Autodesk Fusion 360 part; units mm, degrees
note: some values were not read from the file. Set by a fixed rule: which sketch regions a step uses.
(part 2 of 3)
  arc A385 (-20.318, -125.058) -> (-9.818, -135.558) centre (-9.818, -125.058) ccw
  line L386 (-9.818, -135.558) -> (410.182, -135.558)
  arc A386 (410.182, -135.558) -> (420.682, -125.058) centre (410.182, -125.058) ccw
  line L387 (420.682, -125.058) -> (420.682, 4.942)
  arc A387 (420.682, 4.942) -> (410.182, 15.442) centre (410.182, 4.942) ccw
  line L388 (-20.318, 4.692) -> (-22.818, 4.692)
  line L389 (-23.818, 3.692) -> (-23.818, -4.308)
  line L390 (-22.818, -5.308) -> (-20.318, -5.308)
  line L391 (-20.318, -5.308) -> (-20.318, 4.692)
  arc A388 (-22.818, 4.692) -> (-23.818, 3.692) centre (-22.818, 3.692) ccw
  arc A389 (-23.818, -4.308) -> (-22.818, -5.308) centre (-22.818, -4.308) ccw
  line L392 (-23.818, -26.183) -> (-23.818, -34.183)
  line L393 (-20.318, -25.183) -> (-22.818, -25.183)
  line L394 (-22.818, -35.183) -> (-20.318, -35.183)
  arc A390 (-23.818, -34.183) -> (-22.818, -35.183) centre (-22.818, -34.183) ccw
  arc A391 (-22.818, -25.183) -> (-23.818, -26.183) centre (-22.818, -26.183) ccw
  line L395 (-23.818, -56.058) -> (-23.818, -64.058)
  line L396 (-20.318, -55.058) -> (-22.818, -55.058)
  line L397 (-22.818, -65.058) -> (-20.318, -65.058)
  arc A392 (-23.818, -64.058) -> (-22.818, -65.058) centre (-22.818, -64.058) ccw
  arc A393 (-22.818, -55.058) -> (-23.818, -56.058) centre (-22.818, -56.058) ccw
  line L398 (-23.818, -85.933) -> (-23.818, -93.933)
  line L399 (-20.318, -84.933) -> (-22.818, -84.933)
  line L400 (-22.818, -94.933) -> (-20.318, -94.933)
  arc A394 (-23.818, -93.933) -> (-22.818, -94.933) centre (-22.818, -93.933) ccw
  arc A395 (-22.818, -84.933) -> (-23.818, -85.933) centre (-22.818, -85.933) ccw
  line L401 (-23.818, -115.808) -> (-23.818, -123.808)
  line L402 (-20.318, -114.808) -> (-22.818, -114.808)
  line L403 (-22.818, -124.808) -> (-20.318, -124.808)
  arc A396 (-23.818, -123.808) -> (-22.818, -124.808) centre (-22.818, -123.808) ccw
  arc A397 (-22.818, -114.808) -> (-23.818, -115.808) centre (-22.818, -115.808) ccw
  line L404 (420.682, 4.692) -> (423.182, 4.692)
  line L405 (424.182, 3.692) -> (424.182, -4.308)
  line L406 (423.182, -5.308) -> (420.682, -5.308)
  line L407 (420.682, -5.308) -> (420.682, 4.692)
  arc A398 (424.182, 3.692) -> (423.182, 4.692) centre (423.182, 3.692) ccw
  arc A399 (423.182, -5.308) -> (424.182, -4.308) centre (423.182, -4.308) ccw
  arc A400 (423.182, -65.058) -> (424.182, -64.058) centre (423.182, -64.058) ccw
  line L408 (423.182, -65.058) -> (420.682, -65.058)
  line L409 (424.182, -56.058) -> (424.182, -64.058)
  line L410 (420.682, -55.058) -> (423.182, -55.058)
  arc A401 (424.182, -56.058) -> (423.182, -55.058) centre (423.182, -56.058) ccw
  arc A402 (423.182, -94.933) -> (424.182, -93.933) centre (423.182, -93.933) ccw
  line L411 (423.182, -94.933) -> (420.682, -94.933)
  line L412 (424.182, -85.933) -> (424.182, -93.933)
  line L413 (420.682, -84.933) -> (423.182, -84.933)
  arc A403 (424.182, -85.933) -> (423.182, -84.933) centre (423.182, -85.933) ccw
  line L414 (-9.568, 15.442) -> (0.432, 15.442)
  line L415 (0.432, 15.442) -> (0.432, 17.942)
  line L416 (-0.568, 18.942) -> (-8.568, 18.942)
  line L417 (-9.568, 17.942) -> (-9.568, 15.442)
  arc A404 (-8.568, 18.942) -> (-9.568, 17.942) centre (-8.568, 17.942) ccw
  arc A405 (0.432, 17.942) -> (-0.568, 18.942) centre (-0.568, 17.942) ccw
  line L418 (41.6195, 17.942) -> (41.6195, 15.442)
  arc A406 (42.6195, 18.942) -> (41.6195, 17.942) centre (42.6195, 17.942) ccw
  line L419 (50.6195, 18.942) -> (42.6195, 18.942)
  line L420 (51.6195, 15.442) -> (51.6195, 17.942)
  arc A407 (51.6195, 17.942) -> (50.6195, 18.942) centre (50.6195, 17.942) ccw
  line L421 (92.807, 17.942) -> (92.807, 15.442)
  arc A408 (93.807, 18.942) -> (92.807, 17.942) centre (93.807, 17.942) ccw
  line L422 (101.807, 18.942) -> (93.807, 18.942)
  line L423 (102.807, 15.442) -> (102.807, 17.942)
  arc A409 (102.807, 17.942) -> (101.807, 18.942) centre (101.807, 17.942) ccw
  line L424 (143.9945, 17.942) -> (143.9945, 15.442)
  arc A410 (144.9945, 18.942) -> (143.9945, 17.942) centre (144.9945, 17.942) ccw
  line L425 (152.9945, 18.942) -> (144.9945, 18.942)
  line L426 (153.9945, 15.442) -> (153.9945, 17.942)
  arc A411 (153.9945, 17.942) -> (152.9945, 18.942) centre (152.9945, 17.942) ccw
  line L427 (195.182, 17.942) -> (195.182, 15.442)
  arc A412 (196.182, 18.942) -> (195.182, 17.942) centre (196.182, 17.942) ccw
  line L428 (204.182, 18.942) -> (196.182, 18.942)
  line L429 (205.182, 15.442) -> (205.182, 17.942)
  arc A413 (205.182, 17.942) -> (204.182, 18.942) centre (204.182, 17.942) ccw
  line L430 (246.3695, 17.942) -> (246.3695, 15.442)
  arc A414 (247.3695, 18.942) -> (246.3695, 17.942) centre (247.3695, 17.942) ccw
  line L431 (255.3695, 18.942) -> (247.3695, 18.942)
  line L432 (256.3695, 15.442) -> (256.3695, 17.942)
  arc A415 (256.3695, 17.942) -> (255.3695, 18.942) centre (255.3695, 17.942) ccw
  line L433 (297.557, 17.942) -> (297.557, 15.442)
  arc A416 (298.557, 18.942) -> (297.557, 17.942) centre (298.557, 17.942) ccw
  line L434 (306.557, 18.942) -> (298.557, 18.942)
  line L435 (307.557, 15.442) -> (307.557, 17.942)
  arc A417 (307.557, 17.942) -> (306.557, 18.942) centre (306.557, 17.942) ccw
  line L436 (348.7445, 17.942) -> (348.7445, 15.442)
  arc A418 (349.7445, 18.942) -> (348.7445, 17.942) centre (349.7445, 17.942) ccw
  line L437 (357.7445, 18.942) -> (349.7445, 18.942)
  line L438 (358.7445, 15.442) -> (358.7445, 17.942)
  arc A419 (358.7445, 17.942) -> (357.7445, 18.942) centre (357.7445, 17.942) ccw
  line L439 (399.932, 17.942) -> (399.932, 15.442)
  arc A420 (400.932, 18.942) -> (399.932, 17.942) centre (400.932, 17.942) ccw
  line L440 (408.932, 18.942) -> (400.932, 18.942)
  line L441 (409.932, 15.442) -> (409.932, 17.942)
  arc A421 (409.932, 17.942) -> (408.932, 18.942) centre (408.932, 17.942) ccw
  line L442 (-9.568, -139.4053) -> (-9.818, -139.4053)
  line L443 (-9.568, -135.558) -> (0.432, -135.558)
  line L444 (0.432, -135.558) -> (0.432, -138.058)
  line L445 (-0.568, -139.058) -> (-8.568, -139.058)
  line L446 (-9.568, -138.058) -> (-9.568, -135.558)
  arc A422 (-9.568, -138.058) -> (-8.568, -139.058) centre (-8.568, -138.058) ccw
  arc A423 (-0.568, -139.058) -> (0.432, -138.058) centre (-0.568, -138.058) ccw
  line L447 (41.6195, -138.058) -> (41.6195, -135.558)
  arc A424 (41.6195, -138.058) -> (42.6195, -139.058) centre (42.6195, -138.058) ccw
  line L448 (50.6195, -139.058) -> (42.6195, -139.058)
  arc A425 (50.6195, -139.058) -> (51.6195, -138.058) centre (50.6195, -138.058) ccw
  line L449 (51.6195, -135.558) -> (51.6195, -138.058)
  line L450 (92.807, -138.058) -> (92.807, -135.558)
  arc A426 (92.807, -138.058) -> (93.807, -139.058) centre (93.807, -138.058) ccw
  line L451 (101.807, -139.058) -> (93.807, -139.058)
  arc A427 (101.807, -139.058) -> (102.807, -138.058) centre (101.807, -138.058) ccw
  line L452 (102.807, -135.558) -> (102.807, -138.058)
  line L453 (143.9945, -138.058) -> (143.9945, -135.558)
  arc A428 (143.9945, -138.058) -> (144.9945, -139.058) centre (144.9945, -138.058) ccw
  line L454 (152.9945, -139.058) -> (144.9945, -139.058)
  arc A429 (152.9945, -139.058) -> (153.9945, -138.058) centre (152.9945, -138.058) ccw
  line L455 (153.9945, -135.558) -> (153.9945, -138.058)
  line L456 (195.182, -138.058) -> (195.182, -135.558)
  arc A430 (195.182, -138.058) -> (196.182, -139.058) centre (196.182, -138.058) ccw
  line L457 (204.182, -139.058) -> (196.182, -139.058)
  arc A431 (204.182, -139.058) -> (205.182, -138.058) centre (204.182, -138.058) ccw
  line L458 (205.182, -135.558) -> (205.182, -138.058)
  line L459 (246.3695, -138.058) -> (246.3695, -135.558)
  arc A432 (246.3695, -138.058) -> (247.3695, -139.058) centre (247.3695, -138.058) ccw
  line L460 (255.3695, -139.058) -> (247.3695, -139.058)
  arc A433 (255.3695, -139.058) -> (256.3695, -138.058) centre (255.3695, -138.058) ccw
  line L461 (256.3695, -135.558) -> (256.3695, -138.058)
  line L462 (297.557, -138.058) -> (297.557, -135.558)
  arc A434 (297.557, -138.058) -> (298.557, -139.058) centre (298.557, -138.058) ccw
  line L463 (306.557, -139.058) -> (298.557, -139.058)
  arc A435 (306.557, -139.058) -> (307.557, -138.058) centre (306.557, -138.058) ccw
  line L464 (307.557, -135.558) -> (307.557, -138.058)
  line L465 (348.7445, -138.058) -> (348.7445, -135.558)
  arc A436 (348.7445, -138.058) -> (349.7445, -139.058) centre (349.7445, -138.058) ccw
  line L466 (357.7445, -139.058) -> (349.7445, -139.058)
  arc A437 (357.7445, -139.058) -> (358.7445, -138.058) centre (357.7445, -138.058) ccw
  line L467 (358.7445, -135.558) -> (358.7445, -138.058)
  line L468 (399.932, -138.058) -> (399.932, -135.558)
  arc A438 (399.932, -138.058) -> (400.932, -139.058) centre (400.932, -138.058) ccw
  line L469 (408.932, -139.058) -> (400.932, -139.058)
  arc A439 (408.932, -139.058) -> (409.932, -138.058) centre (408.932, -138.058) ccw
  line L470 (409.932, -135.558) -> (409.932, -138.058)
  arc A440 (373.352, -130.228) -> (376.152, -127.428) centre (373.352, -127.428) ccw
  line L471 (376.152, -125.488) -> (376.152, -127.428)
  arc A441 (376.152, -125.488) -> (373.352, -122.688) centre (373.352, -125.488) ccw
  line L472 (348.552, -122.688) -> (373.352, -122.688)
  arc A442 (348.552, -122.688) -> (345.752, -125.488) centre (348.552, -125.488) ccw
  line L473 (345.752, -127.428) -> (345.752, -125.488)
  arc A443 (345.752, -127.428) -> (348.552, -130.228) centre (348.552, -127.428) ccw
  line L474 (373.352, -130.228) -> (348.552, -130.228)
  arc A444 (395.862, -124.298) -> (394.562, -125.598) centre (395.862, -125.598) ccw
  line L475 (394.562, -130.078) -> (394.562, -125.598)
  arc A445 (394.562, -130.078) -> (395.862, -131.378) centre (395.862, -130.078) ccw
  line L476 (397.802, -131.378) -> (395.862, -131.378)
  arc A446 (397.802, -131.378) -> (399.102, -130.078) centre (397.802, -130.078) ccw
  line L477 (399.102, -125.598) -> (399.102, -130.078)
  arc A447 (399.102, -125.598) -> (397.802, -124.298) centre (397.802, -125.598) ccw
  line L478 (395.862, -124.298) -> (397.802, -124.298)
  arc A448 (383.062, -9.148) -> (381.762, -7.848) centre (381.762, -9.148) ccw
  line L479 (367.122, -7.848) -> (381.762, -7.848)
  arc A449 (367.122, -7.848) -> (365.822, -9.148) centre (367.122, -9.148) ccw
  line L480 (365.822, -13.628) -> (365.822, -9.148)
  arc A450 (365.822, -13.628) -> (367.122, -14.928) centre (367.122, -13.628) ccw
  line L481 (381.762, -14.928) -> (367.122, -14.928)
  arc A451 (381.762, -14.928) -> (383.062, -13.628) centre (381.762, -13.628) ccw
  line L482 (383.062, -9.148) -> (383.062, -13.628)
  line L483 (411.977, -14.103) -> (397.337, -14.103)
  line L484 (396.037, -12.803) -> (396.037, -10.863)
  line L485 (397.337, -9.563) -> (411.977, -9.563)
  arc A452 (396.037, -12.803) -> (397.337, -14.103) centre (397.337, -12.803) ccw
  arc A453 (397.337, -9.563) -> (396.037, -10.863) centre (397.337, -10.863) ccw
  arc A454 (411.977, -14.103) -> (413.277, -12.803) centre (411.977, -12.803) ccw
  line L486 (413.277, -10.863) -> (413.277, -12.803)
  arc A455 (413.277, -10.863) -> (411.977, -9.563) centre (411.977, -10.863) ccw
  arc A456 (412.123, 3.662) -> (410.823, 4.962) centre (410.823, 3.662) ccw
  line L487 (406.143, 4.962) -> (410.823, 4.962)
  arc A457 (406.143, 4.962) -> (404.843, 3.662) centre (406.143, 3.662) ccw
  line L488 (404.843, 1.722) -> (404.843, 3.662)
  arc A458 (404.843, 1.722) -> (406.143, 0.422) centre (406.143, 1.722) ccw
  line L489 (410.823, 0.422) -> (406.143, 0.422)
  arc A459 (410.823, 0.422) -> (412.123, 1.722) centre (410.823, 1.722) ccw
  line L490 (412.123, 3.662) -> (412.123, 1.722)
  point P0 (-23.818, 4.692)
  point P1 (424.182, 4.692)
  point P2 (-9.568, 18.942)
  point P3 (-9.568, -139.058)
  dimension "d12" = 3.5
  dimension "d13" = 10
  dimension "d14" = 1
  dimension "d17" = 0
  dimension "d18" = -119.5
  dimension "d23" = 3.5
  dimension "d24" = 10
  dimension "d25" = 1
  dimension "d28" = 0
  dimension "d29" = -119.5
  dimension "d31" = 10
  dimension "d32" = 3.5
  dimension "d33" = 1
  dimension "d36" = 409.5
  dimension "d37" = 0
  dimension "d39" = 10
  dimension "d40" = 3.5
  dimension "d41" = 1
  dimension "d44" = 409.5
  dimension "d45" = 0
  constraint horizontal L388
  constraint vertical L389
  constraint horizontal L390
  constraint vertical L391
  constraint coincident P0 L388
  constraint coincident P0 L389
  constraint tangent L388 A388
  constraint tangent L389 A388
  constraint tangent L390 A389
  constraint tangent L389 A389
  constraint equal A388 A389
  constraint horizontal L404
  constraint vertical L405
  constraint horizontal L406
  constraint vertical L407
  constraint coincident P1 L404
  constraint coincident P1 L405
  constraint tangent L404 A398
  constraint tangent L405 A398
  constraint tangent L405 A399
  constraint tangent L406 A399
  constraint equal A398 A399
  constraint horizontal L414
  constraint vertical L415
  constraint horizontal L416
  constraint vertical L417
  constraint coincident P2 L417
  constraint coincident P2 L416
  constraint tangent L417 A404
  constraint tangent L416 A404
  constraint tangent L415 A405
  constraint tangent L416 A405
  constraint equal A404 A405
  constraint horizontal L442
  constraint horizontal L443
  constraint vertical L444
  constraint horizontal L445
  constraint vertical L446
  constraint coincident P3 L446
  constraint coincident P3 L445
  constraint tangent L446 A422
  constraint tangent L445 A422
  constraint tangent L445 A423
  constraint tangent L444 A423
  constraint equal A422 A423
  measures "d12" distance of L388.start P0
  measures "d13" distance of L388.start L390.end
  measures "d14" radius of A388
  measures "d23" distance of L404.start P1
  measures "d24" distance of L404.start L406.end
  measures "d25" radius of A398
  measures "d31" distance of L414.start L414.end
  measures "d32" distance of L414.start P2
  measures "d33" radius of A404
  measures "d39" distance of L443.start L443.end
  measures "d40" distance of L443.start P3
  measures "d41" radius of A422
extrude "Extrude1" add sketch "Sketch1" along normal blind 1.5 contours L384 A384 L385 A385 L386 A386 L387 A387 L391 L407 L414 L443 | A440 L471 A441 L472 A442 L473 A443 L474 | A444 L475 A445 L476 A446 L477 A447 L478 | A448 L479 A449 L480 A450 L481 A451 L482 | L483 L484 L485 A452 A453 A454 L486 A455 | A456 L487 A457 L488 A458 L489 A459 L490
extrude "Extrude2" add sketch "Sketch1" along normal blind 1.5 contours L385 L388 L389 L390 L391 A388 A389 | L385 L392 L393 L394 A390 A391 | L385 L395 L396 L397 A392 A393 | L385 L398 L399 L400 A394 A395 | L385 L401 L402 L403 A396 A397
extrude "Extrude3" add sketch "Sketch1" along normal blind 1.5 contours L384 L439 A420 L440 L441 A421 | L387 L404 L405 L406 L407 A398 A399 | L384 L436 A418 L437 L438 A419 | L387 A400 L408 L409 L410 A401 | L384 L433 A416 L434 L435 A417 | L387 A402 L411 L412 L413 A403 | L384 L430 A414 L431 L432 A415 | L384 L427 A412 L428 L429 A413 | L386 L468 A438 L469 A439 L470 | L384 L424 A410 L425 L426 A411 | L386 L465 A436 L466 A437 L467 | L384 L421 A408 L422 L423 A409 | L386 L462 A434 L463 A435 L464 | L384 L418 A406 L419 L420 A407 | L386 L459 A432 L460 A433 L461 | L384 L414 L415 L416 L417 A404 A405 | L386 L456 A430 L457 A431 L458 | L386 L453 A428 L454 A429 L455 | L386 L450 A426 L451 A427 L452 | L386 L447 A424 L448 A425 L449 | L386 L443 L444 L445 L446 A422 A423
extrude "Extrude4" cut sketch "Sketch1" along normal blind 3 contours A440 L471 A441 L472 A442 L473 A443 L474
extrude "Extrude5" cut sketch "Sketch1" along normal blind 2 contours A444 L475 A445 L476 A446 L477 A447 L478
extrude "Extrude6" cut sketch "Sketch1" along normal blind 10 contours A448 L479 A449 L480 A450 L481 A451 L482
extrude "Extrude7" cut sketch "Sketch1" along normal blind 15 contours L483 L484 L485 A452 A453 A454 L486 A455
extrude "Extrude8" cut sketch "Sketch1" along normal blind 5 contours A456 L487 A457 L488 A458 L489 A459 L490
sketch "Sketch3" plane through (0, 0, 1.5) normal (0, 0, 1) x (-1, 0, 0)
  line L0 (-406.143, -4.962) -> (-410.823, -4.962)
  arc A0 (-412.123, -3.662) -> (-410.823, -4.962) centre (-410.823, -3.662) ccw
  line L1 (-412.123, -3.662) -> (-412.123, -1.722)
  arc A1 (-410.823, -0.422) -> (-412.123, -1.722) centre (-410.823, -1.722) ccw
  line L2 (-410.823, -0.422) -> (-406.143, -0.422)
  arc A2 (-404.843, -1.722) -> (-406.143, -0.422) centre (-406.143, -1.722) ccw
  line L3 (-404.843, -1.722) -> (-404.843, -3.662)
  arc A3 (-406.143, -4.962) -> (-404.843, -3.662) centre (-406.143, -3.662) ccw
  line L4 (-411.977, 14.103) -> (-397.337, 14.103)
  arc A4 (-396.037, 12.803) -> (-397.337, 14.103) centre (-397.337, 12.803) ccw
  line L5 (-396.037, 12.803) -> (-396.037, 10.863)
  arc A5 (-397.337, 9.563) -> (-396.037, 10.863) centre (-397.337, 10.863) ccw
  line L6 (-397.337, 9.563) -> (-411.977, 9.563)
  arc A6 (-413.277, 10.863) -> (-411.977, 9.563) centre (-411.977, 10.863) ccw
  line L7 (-413.277, 10.863) -> (-413.277, 12.803)
  arc A7 (-411.977, 14.103) -> (-413.277, 12.803) centre (-411.977, 12.803) ccw
  line L8 (-367.122, 7.848) -> (-381.762, 7.848)
  arc A8 (-383.062, 9.148) -> (-381.762, 7.848) centre (-381.762, 9.148) ccw
  line L9 (-383.062, 9.148) -> (-383.062, 13.628)
  arc A9 (-381.762, 14.928) -> (-383.062, 13.628) centre (-381.762, 13.628) ccw
  line L10 (-381.762, 14.928) -> (-367.122, 14.928)
  arc A10 (-365.822, 13.628) -> (-367.122, 14.928) centre (-367.122, 13.628) ccw
  line L11 (-365.822, 13.628) -> (-365.822, 9.148)
  arc A11 (-367.122, 7.848) -> (-365.822, 9.148) centre (-367.122, 9.148) ccw
  line L12 (-394.562, 130.078) -> (-394.562, 125.598)
  arc A12 (-395.862, 124.298) -> (-394.562, 125.598) centre (-395.862, 125.598) ccw
  line L13 (-395.862, 124.298) -> (-397.802, 124.298)
  arc A13 (-399.102, 125.598) -> (-397.802, 124.298) centre (-397.802, 125.598) ccw
  line L14 (-399.102, 125.598) -> (-399.102, 130.078)
  arc A14 (-397.802, 131.378) -> (-399.102, 130.078) centre (-397.802, 130.078) ccw
  line L15 (-397.802, 131.378) -> (-395.862, 131.378)
  arc A15 (-394.562, 130.078) -> (-395.862, 131.378) centre (-395.862, 130.078) ccw
  line L16 (-376.152, 125.488) -> (-376.152, 127.428)
  arc A16 (-373.352, 130.228) -> (-376.152, 127.428) centre (-373.352, 127.428) ccw
  line L17 (-373.352, 130.228) -> (-348.552, 130.228)
  arc A17 (-345.752, 127.428) -> (-348.552, 130.228) centre (-348.552, 127.428) ccw
  line L18 (-345.752, 127.428) -> (-345.752, 125.488)
  arc A18 (-348.552, 122.688) -> (-345.752, 125.488) centre (-348.552, 125.488) ccw
  line L19 (-348.552, 122.688) -> (-373.352, 122.688)
  arc A19 (-376.152, 125.488) -> (-373.352, 122.688) centre (-373.352, 125.488) ccw
  arc A20 (-50.65, 50.15) -> (-50.15, 50.65) centre (-50.65, 50.65) ccw
  line L20 (-50.65, 50.15) -> (-63.65, 50.15)
  arc A21 (-64.15, 50.65) -> (-63.65, 50.15) centre (-63.65, 50.65) ccw
  line L21 (-64.15, 50.65) -> (-64.15, 63.65)
  arc A22 (-63.65, 64.15) -> (-64.15, 63.65) centre (-63.65, 63.65) ccw
  line L22 (-63.65, 64.15) -> (-50.65, 64.15)
  arc A23 (-50.15, 63.65) -> (-50.65, 64.15) centre (-50.65, 63.65) ccw
  line L23 (-50.15, 63.65) -> (-50.15, 50.65)
  arc A24 (-203.05, 50.15) -> (-202.55, 50.65) centre (-203.05, 50.65) ccw
  line L24 (-203.05, 50.15) -> (-216.05, 50.15)
  arc A25 (-216.55, 50.65) -> (-216.05, 50.15) centre (-216.05, 50.65) ccw
  line L25 (-216.55, 50.65) -> (-216.55, 63.65)
  arc A26 (-216.05, 64.15) -> (-216.55, 63.65) centre (-216.05, 63.65) ccw
  line L26 (-216.05, 64.15) -> (-203.05, 64.15)
  arc A27 (-202.55, 63.65) -> (-203.05, 64.15) centre (-203.05, 63.65) ccw
  line L27 (-202.55, 63.65) -> (-202.55, 50.65)
  arc A28 (-107.8, 50.15) -> (-107.3, 50.65) centre (-107.8, 50.65) ccw
  line L28 (-107.8, 50.15) -> (-120.8, 50.15)
  arc A29 (-121.3, 50.65) -> (-120.8, 50.15) centre (-120.8, 50.65) ccw
  line L29 (-121.3, 50.65) -> (-121.3, 63.65)
  arc A30 (-120.8, 64.15) -> (-121.3, 63.65) centre (-120.8, 63.65) ccw
  line L30 (-120.8, 64.15) -> (-107.8, 64.15)
  arc A31 (-107.3, 63.65) -> (-107.8, 64.15) centre (-107.8, 63.65) ccw
  line L31 (-107.3, 63.65) -> (-107.3, 50.65)
  arc A32 (-267.3438, 107.3) -> (-266.8438, 107.8) centre (-267.3438, 107.8) ccw
  line L32 (-267.3438, 107.3) -> (-280.3438, 107.3)
  arc A33 (-280.8438, 107.8) -> (-280.3438, 107.3) centre (-280.3438, 107.8) ccw
  line L33 (-280.8438, 107.8) -> (-280.8438, 120.8)
  arc A34 (-280.3438, 121.3) -> (-280.8438, 120.8) centre (-280.3438, 120.8) ccw
  line L34 (-280.3438, 121.3) -> (-267.3438, 121.3)
  arc A35 (-266.8438, 120.8) -> (-267.3438, 121.3) centre (-267.3438, 120.8) ccw
  line L35 (-266.8438, 120.8) -> (-266.8438, 107.8)
  arc A36 (-164.95, 2.525) -> (-164.45, 3.025) centre (-164.95, 3.025) ccw
  line L36 (-164.95, 2.525) -> (-177.95, 2.525)
  arc A37 (-178.45, 3.025) -> (-177.95, 2.525) centre (-177.95, 3.025) ccw
  line L37 (-178.45, 3.025) -> (-178.45, 16.025)
  arc A38 (-177.95, 16.525) -> (-178.45, 16.025) centre (-177.95, 16.025) ccw
  line L38 (-177.95, 16.525) -> (-164.95, 16.525)
  arc A39 (-164.45, 16.025) -> (-164.95, 16.525) centre (-164.95, 16.025) ccw
  line L39 (-164.45, 16.025) -> (-164.45, 3.025)
  arc A40 (-60.175, 31.1) -> (-59.675, 31.6) centre (-60.175, 31.6) ccw
  line L40 (-60.175, 31.1) -> (-73.175, 31.1)
  arc A41 (-73.675, 31.6) -> (-73.175, 31.1) centre (-73.175, 31.6) ccw
  line L41 (-73.675, 31.6) -> (-73.675, 44.6)
  arc A42 (-73.175, 45.1) -> (-73.675, 44.6) centre (-73.175, 44.6) ccw
  line L42 (-73.175, 45.1) -> (-60.175, 45.1)
  arc A43 (-59.675, 44.6) -> (-60.175, 45.1) centre (-60.175, 44.6) ccw
  line L43 (-59.675, 44.6) -> (-59.675, 31.6)
  arc A44 (-212.575, 31.1) -> (-212.075, 31.6) centre (-212.575, 31.6) ccw
  line L44 (-212.575, 31.1) -> (-225.575, 31.1)
  arc A45 (-226.075, 31.6) -> (-225.575, 31.1) centre (-225.575, 31.6) ccw
  line L45 (-226.075, 31.6) -> (-226.075, 44.6)
  arc A46 (-225.575, 45.1) -> (-226.075, 44.6) centre (-225.575, 44.6) ccw
  line L46 (-225.575, 45.1) -> (-212.575, 45.1)
  arc A47 (-212.075, 44.6) -> (-212.575, 45.1) centre (-212.575, 44.6) ccw
  line L47 (-212.075, 44.6) -> (-212.075, 31.6)
  arc A48 (-10.1687, 69.2) -> (-9.6687, 69.7) centre (-10.1687, 69.7) ccw
  line L48 (-10.1687, 69.2) -> (-23.1687, 69.2)
  arc A49 (-23.6687, 69.7) -> (-23.1687, 69.2) centre (-23.1688, 69.7) ccw
  line L49 (-23.6687, 69.7) -> (-23.6687, 82.7)
  arc A50 (-23.1687, 83.2) -> (-23.6687, 82.7) centre (-23.1688, 82.7) ccw
  line L50 (-23.1687, 83.2) -> (-10.1687, 83.2)
  arc A51 (-9.6687, 82.7) -> (-10.1687, 83.2) centre (-10.1688, 82.7) ccw
  line L51 (-9.6687, 82.7) -> (-9.6687, 69.7)
  arc A52 (-74.4625, 69.2) -> (-73.9625, 69.7) centre (-74.4625, 69.7) ccw
  line L52 (-74.4625, 69.2) -> (-87.4625, 69.2)
  arc A53 (-87.9625, 69.7) -> (-87.4625, 69.2) centre (-87.4625, 69.7) ccw
  line L53 (-87.9625, 69.7) -> (-87.9625, 82.7)
  arc A54 (-87.4625, 83.2) -> (-87.9625, 82.7) centre (-87.4625, 82.7) ccw
  line L54 (-87.4625, 83.2) -> (-74.4625, 83.2)
  arc A55 (-73.9625, 82.7) -> (-74.4625, 83.2) centre (-74.4625, 82.7) ccw
  line L55 (-73.9625, 82.7) -> (-73.9625, 69.7)
  arc A56 (-245.9125, 69.2) -> (-245.4125, 69.7) centre (-245.9125, 69.7) ccw
  line L56 (-245.9125, 69.2) -> (-258.9125, 69.2)
  arc A57 (-259.4125, 69.7) -> (-258.9125, 69.2) centre (-258.9125, 69.7) ccw
  line L57 (-259.4125, 69.7) -> (-259.4125, 82.7)
  arc A58 (-258.9125, 83.2) -> (-259.4125, 82.7) centre (-258.9125, 82.7) ccw
  line L58 (-258.9125, 83.2) -> (-245.9125, 83.2)
  arc A59 (-245.4125, 82.7) -> (-245.9125, 83.2) centre (-245.9125, 82.7) ccw
  line L59 (-245.4125, 82.7) -> (-245.4125, 69.7)
  arc A60 (-122.0875, 88.25) -> (-121.5875, 88.75) centre (-122.0875, 88.75) ccw
  line L60 (-122.0875, 88.25) -> (-135.0875, 88.25)
  arc A61 (-135.5875, 88.75) -> (-135.0875, 88.25) centre (-135.0875, 88.75) ccw
  line L61 (-135.5875, 88.75) -> (-135.5875, 101.75)
  arc A62 (-135.0875, 102.25) -> (-135.5875, 101.75) centre (-135.0875, 101.75) ccw
  line L62 (-135.0875, 102.25) -> (-122.0875, 102.25)
  arc A63 (-121.5875, 101.75) -> (-122.0875, 102.25) centre (-122.0875, 101.75) ccw
  line L63 (-121.5875, 101.75) -> (-121.5875, 88.75)
  arc A64 (-188.7625, 69.2) -> (-188.2625, 69.7) centre (-188.7625, 69.7) ccw
  line L64 (-188.7625, 69.2) -> (-201.7625, 69.2)
  arc A65 (-202.2625, 69.7) -> (-201.7625, 69.2) centre (-201.7625, 69.7) ccw
  line L65 (-202.2625, 69.7) -> (-202.2625, 82.7)
  arc A66 (-201.7625, 83.2) -> (-202.2625, 82.7) centre (-201.7625, 82.7) ccw
  line L66 (-201.7625, 83.2) -> (-188.7625, 83.2)
  arc A67 (-188.2625, 82.7) -> (-188.7625, 83.2) centre (-188.7625, 82.7) ccw
  line L67 (-188.2625, 82.7) -> (-188.2625, 69.7)
  arc A68 (-117.325, 31.1) -> (-116.825, 31.6) centre (-117.325, 31.6) ccw
  line L68 (-117.325, 31.1) -> (-130.325, 31.1)
  arc A69 (-130.825, 31.6) -> (-130.325, 31.1) centre (-130.325, 31.6) ccw
  line L69 (-130.825, 31.6) -> (-130.825, 44.6)
  arc A70 (-130.325, 45.1) -> (-130.825, 44.6) centre (-130.325, 44.6) ccw
  line L70 (-130.325, 45.1) -> (-117.325, 45.1)
  arc A71 (-116.825, 44.6) -> (-117.325, 45.1) centre (-117.325, 44.6) ccw
  line L71 (-116.825, 44.6) -> (-116.825, 31.6)
  arc A72 (-312.5875, 88.25) -> (-312.0875, 88.75) centre (-312.5875, 88.75) ccw
  line L72 (-312.5875, 88.25) -> (-325.5875, 88.25)
  arc A73 (-326.0875, 88.75) -> (-325.5875, 88.25) centre (-325.5875, 88.75) ccw
  line L73 (-326.0875, 88.75) -> (-326.0875, 101.75)
  arc A74 (-325.5875, 102.25) -> (-326.0875, 101.75) centre (-325.5875, 101.75) ccw
  line L74 (-325.5875, 102.25) -> (-312.5875, 102.25)
  arc A75 (-312.0875, 101.75) -> (-312.5875, 102.25) centre (-312.5875, 101.75) ccw
  line L75 (-312.0875, 101.75) -> (-312.0875, 88.75)
  arc A76 (-169.7125, 69.2) -> (-169.2125, 69.7) centre (-169.7125, 69.7) ccw
  line L76 (-169.7125, 69.2) -> (-182.7125, 69.2)
  arc A77 (-183.2125, 69.7) -> (-182.7125, 69.2) centre (-182.7125, 69.7) ccw
  line L77 (-183.2125, 69.7) -> (-183.2125, 82.7)
  arc A78 (-182.7125, 83.2) -> (-183.2125, 82.7) centre (-182.7125, 82.7) ccw
  line L78 (-182.7125, 83.2) -> (-169.7125, 83.2)
  arc A79 (-169.2125, 82.7) -> (-169.7125, 83.2) centre (-169.7125, 82.7) ccw
  line L79 (-169.2125, 82.7) -> (-169.2125, 69.7)
  arc A80 (-219.7188, 107.3) -> (-219.2188, 107.8) centre (-219.7187, 107.8) ccw
  line L80 (-219.7188, 107.3) -> (-232.7188, 107.3)
  arc A81 (-233.2188, 107.8) -> (-232.7188, 107.3) centre (-232.7188, 107.8) ccw
  line L81 (-233.2188, 107.8) -> (-233.2188, 120.8)
  arc A82 (-232.7188, 121.3) -> (-233.2188, 120.8) centre (-232.7188, 120.8) ccw
  line L82 (-232.7188, 121.3) -> (-219.7188, 121.3)
  arc A83 (-219.2188, 120.8) -> (-219.7188, 121.3) centre (-219.7188, 120.8) ccw
  line L83 (-219.2188, 120.8) -> (-219.2188, 107.8)
  arc A84 (-31.6, 50.15) -> (-31.1, 50.65) centre (-31.6, 50.65) ccw
  line L84 (-31.6, 50.15) -> (-44.6, 50.15)
  arc A85 (-45.1, 50.65) -> (-44.6, 50.15) centre (-44.6, 50.65) ccw
  line L85 (-45.1, 50.65) -> (-45.1, 63.65)
  arc A86 (-44.6, 64.15) -> (-45.1, 63.65) centre (-44.6, 63.65) ccw
  line L86 (-44.6, 64.15) -> (-31.6, 64.15)
  arc A87 (-31.1, 63.65) -> (-31.6, 64.15) centre (-31.6, 63.65) ccw
  line L87 (-31.1, 63.65) -> (-31.1, 50.65)
  arc A88 (-79.225, 2.525) -> (-78.725, 3.025) centre (-79.225, 3.025) ccw
  line L88 (-79.225, 2.525) -> (-92.225, 2.525)
  arc A89 (-92.725, 3.025) -> (-92.225, 2.525) centre (-92.225, 3.025) ccw
  line L89 (-92.725, 3.025) -> (-92.725, 16.025)
  arc A90 (-92.225, 16.525) -> (-92.725, 16.025) centre (-92.225, 16.025) ccw
  line L90 (-92.225, 16.525) -> (-79.225, 16.525)
  arc A91 (-78.725, 16.025) -> (-79.225, 16.525) centre (-79.225, 16.025) ccw
  line L91 (-78.725, 16.025) -> (-78.725, 3.025)
  arc A92 (-226.8625, 69.2) -> (-226.3625, 69.7) centre (-226.8625, 69.7) ccw
  line L92 (-226.8625, 69.2) -> (-239.8625, 69.2)
  arc A93 (-240.3625, 69.7) -> (-239.8625, 69.2) centre (-239.8625, 69.7) ccw
  line L93 (-240.3625, 69.7) -> (-240.3625, 82.7)
  arc A94 (-239.8625, 83.2) -> (-240.3625, 82.7) centre (-239.8625, 82.7) ccw
  line L94 (-239.8625, 83.2) -> (-226.8625, 83.2)
  arc A95 (-226.3625, 82.7) -> (-226.8625, 83.2) centre (-226.8625, 82.7) ccw
  line L95 (-226.3625, 82.7) -> (-226.3625, 69.7)
  arc A96 (-131.6125, 69.2) -> (-131.1125, 69.7) centre (-131.6125, 69.7) ccw
  line L96 (-131.6125, 69.2) -> (-144.6125, 69.2)
  arc A97 (-145.1125, 69.7) -> (-144.6125, 69.2) centre (-144.6125, 69.7) ccw
  line L97 (-145.1125, 69.7) -> (-145.1125, 82.7)
  arc A98 (-144.6125, 83.2) -> (-145.1125, 82.7) centre (-144.6125, 82.7) ccw
  line L98 (-144.6125, 83.2) -> (-131.6125, 83.2)
  arc A99 (-131.1125, 82.7) -> (-131.6125, 83.2) centre (-131.6125, 82.7) ccw
  line L99 (-131.1125, 82.7) -> (-131.1125, 69.7)
  arc A100 (-279.8438, 51.737) -> (-279.3438, 51.237) centre (-279.3438, 51.737) ccw
  line L100 (-279.8438, 51.737) -> (-279.8438, 57.737)
  arc A101 (-279.3438, 58.237) -> (-279.8438, 57.737) centre (-279.3437, 57.737) ccw
  line L101 (-279.3438, 58.237) -> (-265.3438, 58.237)
  arc A102 (-264.8438, 57.737) -> (-265.3438, 58.237) centre (-265.3438, 57.737) ccw
  line L102 (-264.8438, 57.737) -> (-264.8438, 51.737)
  arc A103 (-265.3438, 51.237) -> (-264.8438, 51.737) centre (-265.3438, 51.737) ccw
  line L103 (-265.3438, 51.237) -> (-279.3438, 51.237)
  arc A104 (-251.762, 32.1) -> (-251.262, 32.6) centre (-251.762, 32.6) ccw
  line L104 (-251.762, 32.1) -> (-257.762, 32.1)
  arc A105 (-258.262, 32.6) -> (-257.762, 32.1) centre (-257.762, 32.6) ccw
  line L105 (-258.262, 32.6) -> (-258.262, 46.6)
  arc A106 (-257.762, 47.1) -> (-258.262, 46.6) centre (-257.762, 46.6) ccw
  line L106 (-257.762, 47.1) -> (-251.762, 47.1)
  arc A107 (-251.262, 46.6) -> (-251.762, 47.1) centre (-251.762, 46.6) ccw
  line L107 (-251.262, 46.6) -> (-251.262, 32.6)
  arc A108 (-268.4943, 89.25) -> (-267.9943, 89.75) centre (-268.4943, 89.75) ccw
  line L108 (-268.4943, 89.25) -> (-274.4943, 89.25)
  arc A109 (-274.9943, 89.75) -> (-274.4943, 89.25) centre (-274.4943, 89.75) ccw
  line L109 (-274.9943, 89.75) -> (-274.9943, 103.75)
  arc A110 (-274.4943, 104.25) -> (-274.9943, 103.75) centre (-274.4943, 103.75) ccw
  line L110 (-274.4943, 104.25) -> (-268.4943, 104.25)
  arc A111 (-267.9943, 103.75) -> (-268.4943, 104.25) centre (-268.4943, 103.75) ccw
  line L111 (-267.9943, 103.75) -> (-267.9943, 89.75)
  arc A112 (-312.5875, 50.15) -> (-312.0875, 50.65) centre (-312.5875, 50.65) ccw
  line L112 (-312.5875, 50.15) -> (-325.5875, 50.15)
  arc A113 (-326.0875, 50.65) -> (-325.5875, 50.15) centre (-325.5875, 50.65) ccw
  line L113 (-326.0875, 50.65) -> (-326.0875, 63.65)
  arc A114 (-325.5875, 64.15) -> (-326.0875, 63.65) centre (-325.5875, 63.65) ccw
  line L114 (-325.5875, 64.15) -> (-312.5875, 64.15)
  arc A115 (-312.0875, 63.65) -> (-312.5875, 64.15) centre (-312.5875, 63.65) ccw
  line L115 (-312.0875, 63.65) -> (-312.0875, 50.65)
  arc A116 (-312.5875, 107.3) -> (-312.0875, 107.8) centre (-312.5875, 107.8) ccw
  line L116 (-312.5875, 107.3) -> (-325.5875, 107.3)
  arc A117 (-326.0875, 107.8) -> (-325.5875, 107.3) centre (-325.5875, 107.8) ccw
  line L117 (-326.0875, 107.8) -> (-326.0875, 120.8)
  arc A118 (-325.5875, 121.3) -> (-326.0875, 120.8) centre (-325.5875, 120.8) ccw
  line L118 (-325.5875, 121.3) -> (-312.5875, 121.3)
  arc A119 (-312.0875, 120.8) -> (-312.5875, 121.3) centre (-312.5875, 120.8) ccw
  line L119 (-312.0875, 120.8) -> (-312.0875, 107.8)
  arc A120 (-98.275, 31.1) -> (-97.775, 31.6) centre (-98.275, 31.6) ccw
  line L120 (-98.275, 31.1) -> (-111.275, 31.1)
  arc A121 (-111.775, 31.6) -> (-111.275, 31.1) centre (-111.275, 31.6) ccw
  line L121 (-111.775, 31.6) -> (-111.775, 44.6)
  arc A122 (-111.275, 45.1) -> (-111.775, 44.6) centre (-111.275, 44.6) ccw
  line L122 (-111.275, 45.1) -> (-98.275, 45.1)
  arc A123 (-97.775, 44.6) -> (-98.275, 45.1) centre (-98.275, 44.6) ccw
  line L123 (-97.775, 44.6) -> (-97.775, 31.6)
  arc A124 (-250.675, 2.525) -> (-250.175, 3.025) centre (-250.675, 3.025) ccw
  line L124 (-250.675, 2.525) -> (-263.675, 2.525)
  arc A125 (-264.175, 3.025) -> (-263.675, 2.525) centre (-263.675, 3.025) ccw
  line L125 (-264.175, 3.025) -> (-264.175, 16.025)
  arc A126 (-263.675, 16.525) -> (-264.175, 16.025) centre (-263.675, 16.025) ccw
  line L126 (-263.675, 16.525) -> (-250.675, 16.525)
  arc A127 (-250.175, 16.025) -> (-250.675, 16.525) centre (-250.675, 16.025) ccw
  line L127 (-250.175, 16.025) -> (-250.175, 3.025)
  arc A128 (-312.5875, 2.525) -> (-312.0875, 3.025) centre (-312.5875, 3.025) ccw
  line L128 (-312.5875, 2.525) -> (-325.5875, 2.525)
  arc A129 (-326.0875, 3.025) -> (-325.5875, 2.525) centre (-325.5875, 3.025) ccw
  line L129 (-326.0875, 3.025) -> (-326.0875, 16.025)
  arc A130 (-325.5875, 16.525) -> (-326.0875, 16.025) centre (-325.5875, 16.025) ccw
  line L130 (-325.5875, 16.525) -> (-312.5875, 16.525)
  arc A131 (-312.0875, 16.025) -> (-312.5875, 16.525) centre (-312.5875, 16.025) ccw
  line L131 (-312.0875, 16.025) -> (-312.0875, 3.025)
  arc A132 (-29.2188, 107.3) -> (-28.7187, 107.8) centre (-29.2188, 107.8) ccw
  line L132 (-29.2188, 107.3) -> (-42.2188, 107.3)
  arc A133 (-42.7188, 107.8) -> (-42.2188, 107.3) centre (-42.2188, 107.8) ccw
  line L133 (-42.7188, 107.8) -> (-42.7188, 120.8)
  arc A134 (-42.2188, 121.3) -> (-42.7188, 120.8) centre (-42.2187, 120.8) ccw
  line L134 (-42.2188, 121.3) -> (-29.2188, 121.3)
  arc A135 (-28.7188, 120.8) -> (-29.2188, 121.3) centre (-29.2187, 120.8) ccw
  line L135 (-28.7188, 120.8) -> (-28.7187, 107.8)
  arc A136 (-124.4688, 107.3) -> (-123.9688, 107.8) centre (-124.4688, 107.8) ccw
  line L136 (-124.4688, 107.3) -> (-137.4688, 107.3)
  arc A137 (-137.9688, 107.8) -> (-137.4688, 107.3) centre (-137.4688, 107.8) ccw
  line L137 (-137.9688, 107.8) -> (-137.9688, 120.8)
  arc A138 (-137.4688, 121.3) -> (-137.9688, 120.8) centre (-137.4687, 120.8) ccw
  line L138 (-137.4688, 121.3) -> (-124.4688, 121.3)
  arc A139 (-123.9688, 120.8) -> (-124.4688, 121.3) centre (-124.4688, 120.8) ccw
  line L139 (-123.9688, 120.8) -> (-123.9688, 107.8)
  arc A140 (-41.125, 31.1) -> (-40.625, 31.6) centre (-41.125, 31.6) ccw
  line L140 (-41.125, 31.1) -> (-54.125, 31.1)
  arc A141 (-54.625, 31.6) -> (-54.125, 31.1) centre (-54.125, 31.6) ccw
  line L141 (-54.625, 31.6) -> (-54.625, 44.6)
  arc A142 (-54.125, 45.1) -> (-54.625, 44.6) centre (-54.125, 44.6) ccw
  line L142 (-54.125, 45.1) -> (-41.125, 45.1)
  arc A143 (-40.625, 44.6) -> (-41.125, 45.1) centre (-41.125, 44.6) ccw
  line L143 (-40.625, 44.6) -> (-40.625, 31.6)
  arc A144 (-293.5375, 31.1) -> (-293.0375, 31.6) centre (-293.5375, 31.6) ccw
  line L144 (-293.5375, 31.1) -> (-306.5375, 31.1)
  arc A145 (-307.0375, 31.6) -> (-306.5375, 31.1) centre (-306.5375, 31.6) ccw
  line L145 (-307.0375, 31.6) -> (-307.0375, 44.6)
  arc A146 (-306.5375, 45.1) -> (-307.0375, 44.6) centre (-306.5375, 44.6) ccw
  line L146 (-306.5375, 45.1) -> (-293.5375, 45.1)
  arc A147 (-293.0375, 44.6) -> (-293.5375, 45.1) centre (-293.5375, 44.6) ccw
  line L147 (-293.0375, 44.6) -> (-293.0375, 31.6)
  arc A148 (-36.3625, 69.2) -> (-35.8625, 69.7) centre (-36.3625, 69.7) ccw
  line L148 (-36.3625, 69.2) -> (-49.3625, 69.2)
  arc A149 (-49.8625, 69.7) -> (-49.3625, 69.2) centre (-49.3625, 69.7) ccw
  line L149 (-49.8625, 69.7) -> (-49.8625, 82.7)
  arc A150 (-49.3625, 83.2) -> (-49.8625, 82.7) centre (-49.3625, 82.7) ccw
  line L150 (-49.3625, 83.2) -> (-36.3625, 83.2)
  arc A151 (-35.8625, 82.7) -> (-36.3625, 83.2) centre (-36.3625, 82.7) ccw
  line L151 (-35.8625, 82.7) -> (-35.8625, 69.7)
  arc A152 (-145.9, 2.525) -> (-145.4, 3.025) centre (-145.9, 3.025) ccw
  line L152 (-145.9, 2.525) -> (-158.9, 2.525)
  arc A153 (-159.4, 3.025) -> (-158.9, 2.525) centre (-158.9, 3.025) ccw
  line L153 (-159.4, 3.025) -> (-159.4, 16.025)
  arc A154 (-158.9, 16.525) -> (-159.4, 16.025) centre (-158.9, 16.025) ccw
  line L154 (-158.9, 16.525) -> (-145.9, 16.525)
  arc A155 (-145.4, 16.025) -> (-145.9, 16.525) centre (-145.9, 16.025) ccw
  line L155 (-145.4, 16.025) -> (-145.4, 3.025)
  arc A156 (-279.8438, 75.613) -> (-279.3438, 75.113) centre (-279.3438, 75.613) ccw
  line L156 (-279.8438, 75.613) -> (-279.8438, 81.613)
  arc A157 (-279.3438, 82.113) -> (-279.8438, 81.613) centre (-279.3438, 81.613) ccw
  line L157 (-279.3438, 82.113) -> (-265.3438, 82.113)
  arc A158 (-264.8438, 81.613) -> (-265.3438, 82.113) centre (-265.3438, 81.613) ccw
  line L158 (-264.8438, 81.613) -> (-264.8438, 75.613)
  arc A159 (-265.3438, 75.113) -> (-264.8437, 75.613) centre (-265.3438, 75.613) ccw
  line L159 (-265.3438, 75.113) -> (-279.3438, 75.113)
  arc A160 (-312.5875, 31.1) -> (-312.0875, 31.6) centre (-312.5875, 31.6) ccw
  line L160 (-312.5875, 31.1) -> (-325.5875, 31.1)
  arc A161 (-326.0875, 31.6) -> (-325.5875, 31.1) centre (-325.5875, 31.6) ccw
  line L161 (-326.0875, 31.6) -> (-326.0875, 44.6)
  arc A162 (-325.5875, 45.1) -> (-326.0875, 44.6) centre (-325.5875, 44.6) ccw
  line L162 (-325.5875, 45.1) -> (-312.5875, 45.1)
  arc A163 (-312.0875, 44.6) -> (-312.5875, 45.1) centre (-312.5875, 44.6) ccw
  line L163 (-312.0875, 44.6) -> (-312.0875, 31.6)
  arc A164 (-293.5375, 107.3) -> (-293.0375, 107.8) centre (-293.5375, 107.8) ccw
  line L164 (-293.5375, 107.3) -> (-306.5375, 107.3)
  arc A165 (-307.0375, 107.8) -> (-306.5375, 107.3) centre (-306.5375, 107.8) ccw
  line L165 (-307.0375, 107.8) -> (-307.0375, 120.8)
  arc A166 (-306.5375, 121.3) -> (-307.0375, 120.8) centre (-306.5375, 120.8) ccw
  line L166 (-306.5375, 121.3) -> (-293.5375, 121.3)
  arc A167 (-293.0375, 120.8) -> (-293.5375, 121.3) centre (-293.5375, 120.8) ccw
  line L167 (-293.0375, 120.8) -> (-293.0375, 107.8)
  arc A168 (-184, 2.525) -> (-183.5, 3.025) centre (-184, 3.025) ccw
  line L168 (-184, 2.525) -> (-197, 2.525)
  arc A169 (-197.5, 3.025) -> (-197, 2.525) centre (-197, 3.025) ccw
  line L169 (-197.5, 3.025) -> (-197.5, 16.025)
  arc A170 (-197, 16.525) -> (-197.5, 16.025) centre (-197, 16.025) ccw
  line L170 (-197, 16.525) -> (-184, 16.525)
  arc A171 (-183.5, 16.025) -> (-184, 16.525) centre (-184, 16.025) ccw
  line L171 (-183.5, 16.025) -> (-183.5, 3.025)
  arc A172 (-231.625, 31.1) -> (-231.125, 31.6) centre (-231.625, 31.6) ccw
  line L172 (-231.625, 31.1) -> (-244.625, 31.1)
  arc A173 (-245.125, 31.6) -> (-244.625, 31.1) centre (-244.625, 31.6) ccw
  line L173 (-245.125, 31.6) -> (-245.125, 44.6)
  arc A174 (-244.625, 45.1) -> (-245.125, 44.6) centre (-244.625, 44.6) ccw
  line L174 (-244.625, 45.1) -> (-231.625, 45.1)
  arc A175 (-231.125, 44.6) -> (-231.625, 45.1) centre (-231.625, 44.6) ccw
  line L175 (-231.125, 44.6) -> (-231.125, 31.6)
  arc A176 (-160.1875, 88.25) -> (-159.6875, 88.75) centre (-160.1875, 88.75) ccw
  line L176 (-160.1875, 88.25) -> (-173.1875, 88.25)
  arc A177 (-173.6875, 88.75) -> (-173.1875, 88.25) centre (-173.1875, 88.75) ccw
  line L177 (-173.6875, 88.75) -> (-173.6875, 101.75)
  arc A178 (-173.1875, 102.25) -> (-173.6875, 101.75) centre (-173.1875, 101.75) ccw
  line L178 (-173.1875, 102.25) -> (-160.1875, 102.25)
  arc A179 (-159.6875, 101.75) -> (-160.1875, 102.25) centre (-160.1875, 101.75) ccw
  line L179 (-159.6875, 101.75) -> (-159.6875, 88.75)
  arc A180 (-98.275, 2.525) -> (-97.775, 3.025) centre (-98.275, 3.025) ccw
  line L180 (-98.275, 2.525) -> (-111.275, 2.525)
  arc A181 (-111.775, 3.025) -> (-111.275, 2.525) centre (-111.275, 3.025) ccw
  line L181 (-111.775, 3.025) -> (-111.775, 16.025)
  arc A182 (-111.275, 16.525) -> (-111.775, 16.025) centre (-111.275, 16.025) ccw
  line L182 (-111.275, 16.525) -> (-98.275, 16.525)
  arc A183 (-97.775, 16.025) -> (-98.275, 16.525) centre (-98.275, 16.025) ccw
  line L183 (-97.775, 16.025) -> (-97.775, 3.025)
  arc A184 (-164.95, 50.15) -> (-164.45, 50.65) centre (-164.95, 50.65) ccw
  line L184 (-164.95, 50.15) -> (-177.95, 50.15)
  arc A185 (-178.45, 50.65) -> (-177.95, 50.15) centre (-177.95, 50.65) ccw
  line L185 (-178.45, 50.65) -> (-178.45, 63.65)
  arc A186 (-177.95, 64.15) -> (-178.45, 63.65) centre (-177.95, 63.65) ccw
  line L186 (-177.95, 64.15) -> (-164.95, 64.15)
  arc A187 (-164.45, 63.65) -> (-164.95, 64.15) centre (-164.95, 63.65) ccw
  line L187 (-164.45, 63.65) -> (-164.45, 50.65)
  arc A188 (-3.025, 2.525) -> (-2.525, 3.025) centre (-3.025, 3.025) ccw
  line L188 (-3.025, 2.525) -> (-16.025, 2.525)
  arc A189 (-16.525, 3.025) -> (-16.025, 2.525) centre (-16.025, 3.025) ccw
  line L189 (-16.525, 3.025) -> (-16.525, 16.025)
  arc A190 (-16.025, 16.525) -> (-16.525, 16.025) centre (-16.025, 16.025) ccw
  line L190 (-16.025, 16.525) -> (-3.025, 16.525)
  arc A191 (-2.525, 16.025) -> (-3.025, 16.525) centre (-3.025, 16.025) ccw
  line L191 (-2.525, 16.025) -> (-2.525, 3.025)
  arc A192 (-45.8875, 88.25) -> (-45.3875, 88.75) centre (-45.8875, 88.75) ccw
  line L192 (-45.8875, 88.25) -> (-58.8875, 88.25)
  arc A193 (-59.3875, 88.75) -> (-58.8875, 88.25) centre (-58.8875, 88.75) ccw
  line L193 (-59.3875, 88.75) -> (-59.3875, 101.75)
  arc A194 (-58.8875, 102.25) -> (-59.3875, 101.75) centre (-58.8875, 101.75) ccw
  line L194 (-58.8875, 102.25) -> (-45.8875, 102.25)
  arc A195 (-45.3875, 101.75) -> (-45.8875, 102.25) centre (-45.8875, 101.75) ccw
  line L195 (-45.3875, 101.75) -> (-45.3875, 88.75)
  arc A196 (-103.0375, 88.25) -> (-102.5375, 88.75) centre (-103.0375, 88.75) ccw
  line L196 (-103.0375, 88.25) -> (-116.0375, 88.25)
  arc A197 (-116.5375, 88.75) -> (-116.0375, 88.25) centre (-116.0375, 88.75) ccw
  line L197 (-116.5375, 88.75) -> (-116.5375, 101.75)
  arc A198 (-116.0375, 102.25) -> (-116.5375, 101.75) centre (-116.0375, 101.75) ccw
  line L198 (-116.0375, 102.25) -> (-103.0375, 102.25)
  arc A199 (-102.5375, 101.75) -> (-103.0375, 102.25) centre (-103.0375, 101.75) ccw
  line L199 (-102.5375, 101.75) -> (-102.5375, 88.75)
  arc A200 (-193.525, 31.1) -> (-193.025, 31.6) centre (-193.525, 31.6) ccw
  line L200 (-193.525, 31.1) -> (-206.525, 31.1)
  arc A201 (-207.025, 31.6) -> (-206.525, 31.1) centre (-206.525, 31.6) ccw
  line L201 (-207.025, 31.6) -> (-207.025, 44.6)
  arc A202 (-206.525, 45.1) -> (-207.025, 44.6) centre (-206.525, 44.6) ccw
  line L202 (-206.525, 45.1) -> (-193.525, 45.1)
  arc A203 (-193.025, 44.6) -> (-193.525, 45.1) centre (-193.525, 44.6) ccw
  line L203 (-193.025, 44.6) -> (-193.025, 31.6)
  arc A204 (-136.375, 31.1) -> (-135.875, 31.6) centre (-136.375, 31.6) ccw
  line L204 (-136.375, 31.1) -> (-149.375, 31.1)
  arc A205 (-149.875, 31.6) -> (-149.375, 31.1) centre (-149.375, 31.6) ccw
  line L205 (-149.875, 31.6) -> (-149.875, 44.6)
  arc A206 (-149.375, 45.1) -> (-149.875, 44.6) centre (-149.375, 44.6) ccw
  line L206 (-149.375, 45.1) -> (-136.375, 45.1)
  arc A207 (-135.875, 44.6) -> (-136.375, 45.1) centre (-136.375, 44.6) ccw
  line L207 (-135.875, 44.6) -> (-135.875, 31.6)
  arc A208 (-93.5125, 69.2) -> (-93.0125, 69.7) centre (-93.5125, 69.7) ccw
  line L208 (-93.5125, 69.2) -> (-106.5125, 69.2)
  arc A209 (-107.0125, 69.7) -> (-106.5125, 69.2) centre (-106.5125, 69.7) ccw
  line L209 (-107.0125, 69.7) -> (-107.0125, 82.7)
  arc A210 (-106.5125, 83.2) -> (-107.0125, 82.7) centre (-106.5125, 82.7) ccw
  line L210 (-106.5125, 83.2) -> (-93.5125, 83.2)
  arc A211 (-93.0125, 82.7) -> (-93.5125, 83.2) centre (-93.5125, 82.7) ccw
  line L211 (-93.0125, 82.7) -> (-93.0125, 69.7)
  arc A212 (-331.6375, 50.15) -> (-331.1375, 50.65) centre (-331.6375, 50.65) ccw
  line L212 (-331.6375, 50.15) -> (-344.6375, 50.15)
  arc A213 (-345.1375, 50.65) -> (-344.6375, 50.15) centre (-344.6375, 50.65) ccw
  line L213 (-345.1375, 50.65) -> (-345.1375, 63.65)
  arc A214 (-344.6375, 64.15) -> (-345.1375, 63.65) centre (-344.6375, 63.65) ccw
  line L214 (-344.6375, 64.15) -> (-331.6375, 64.15)
  arc A215 (-331.1375, 63.65) -> (-331.6375, 64.15) centre (-331.6375, 63.65) ccw
  line L215 (-331.1375, 63.65) -> (-331.1375, 50.65)
  arc A216 (-41.125, 2.525) -> (-40.625, 3.025) centre (-41.125, 3.025) ccw
  line L216 (-41.125, 2.525) -> (-54.125, 2.525)
  arc A217 (-54.625, 3.025) -> (-54.125, 2.525) centre (-54.125, 3.025) ccw
  line L217 (-54.625, 3.025) -> (-54.625, 16.025)
  arc A218 (-54.125, 16.525) -> (-54.625, 16.025) centre (-54.125, 16.025) ccw
  line L218 (-54.125, 16.525) -> (-41.125, 16.525)
  arc A219 (-40.625, 16.025) -> (-41.125, 16.525) centre (-41.125, 16.025) ccw
  line L219 (-40.625, 16.025) -> (-40.625, 3.025)
  arc A220 (-222.1, 50.15) -> (-221.6, 50.65) centre (-222.1, 50.65) ccw
  line L220 (-222.1, 50.15) -> (-235.1, 50.15)
  arc A221 (-235.6, 50.65) -> (-235.1, 50.15) centre (-235.1, 50.65) ccw
  line L221 (-235.6, 50.65) -> (-235.6, 63.65)
  arc A222 (-235.1, 64.15) -> (-235.6, 63.65) centre (-235.1, 63.65) ccw
  line L222 (-235.1, 64.15) -> (-222.1, 64.15)
  arc A223 (-221.6, 63.65) -> (-222.1, 64.15) centre (-222.1, 63.65) ccw
  line L223 (-221.6, 63.65) -> (-221.6, 50.65)
  arc A224 (-7.7875, 50.15) -> (-7.2875, 50.65) centre (-7.7875, 50.65) ccw
  line L224 (-7.7875, 50.15) -> (-20.7875, 50.15)
  arc A225 (-21.2875, 50.65) -> (-20.7875, 50.15) centre (-20.7875, 50.65) ccw
  line L225 (-21.2875, 50.65) -> (-21.2875, 63.65)
  arc A226 (-20.7875, 64.15) -> (-21.2875, 63.65) centre (-20.7875, 63.65) ccw
  line L226 (-20.7875, 64.15) -> (-7.7875, 64.15)
  arc A227 (-7.2875, 63.65) -> (-7.7875, 64.15) centre (-7.7875, 63.65) ccw
  line L227 (-7.2875, 63.65) -> (-7.2875, 50.65)
  arc A228 (-207.8125, 69.2) -> (-207.3125, 69.7) centre (-207.8125, 69.7) ccw
  line L228 (-207.8125, 69.2) -> (-220.8125, 69.2)
  arc A229 (-221.3125, 69.7) -> (-220.8125, 69.2) centre (-220.8125, 69.7) ccw
  line L229 (-221.3125, 69.7) -> (-221.3125, 82.7)
  arc A230 (-220.8125, 83.2) -> (-221.3125, 82.7) centre (-220.8125, 82.7) ccw
  line L230 (-220.8125, 83.2) -> (-207.8125, 83.2)
  arc A231 (-207.3125, 82.7) -> (-207.8125, 83.2) centre (-207.8125, 82.7) ccw
  line L231 (-207.3125, 82.7) -> (-207.3125, 69.7)
  arc A232 (-179.2375, 88.25) -> (-178.7375, 88.75) centre (-179.2375, 88.75) ccw
  line L232 (-179.2375, 88.25) -> (-192.2375, 88.25)
  arc A233 (-192.7375, 88.75) -> (-192.2375, 88.25) centre (-192.2375, 88.75) ccw
  line L233 (-192.7375, 88.75) -> (-192.7375, 101.75)
  arc A234 (-192.2375, 102.25) -> (-192.7375, 101.75) centre (-192.2375, 101.75) ccw
  line L234 (-192.2375, 102.25) -> (-179.2375, 102.25)
  arc A235 (-178.7375, 101.75) -> (-179.2375, 102.25) centre (-179.2375, 101.75) ccw
  line L235 (-178.7375, 101.75) -> (-178.7375, 88.75)
  arc A236 (-150.6625, 69.2) -> (-150.1625, 69.7) centre (-150.6625, 69.7) ccw
  line L236 (-150.6625, 69.2) -> (-163.6625, 69.2)
  arc A237 (-164.1625, 69.7) -> (-163.6625, 69.2) centre (-163.6625, 69.7) ccw
  line L237 (-164.1625, 69.7) -> (-164.1625, 82.7)
  arc A238 (-163.6625, 83.2) -> (-164.1625, 82.7) centre (-163.6625, 82.7) ccw
  line L238 (-163.6625, 83.2) -> (-150.6625, 83.2)
  arc A239 (-150.1625, 82.7) -> (-150.6625, 83.2) centre (-150.6625, 82.7) ccw
  line L239 (-150.1625, 82.7) -> (-150.1625, 69.7)
  arc A240 (-26.8375, 88.25) -> (-26.3375, 88.75) centre (-26.8375, 88.75) ccw
  line L240 (-26.8375, 88.25) -> (-39.8375, 88.25)
  arc A241 (-40.3375, 88.75) -> (-39.8375, 88.25) centre (-39.8375, 88.75) ccw
  line L241 (-40.3375, 88.75) -> (-40.3375, 101.75)
  arc A242 (-39.8375, 102.25) -> (-40.3375, 101.75) centre (-39.8375, 101.75) ccw
  line L242 (-39.8375, 102.25) -> (-26.8375, 102.25)
  arc A243 (-26.3375, 101.75) -> (-26.8375, 102.25) centre (-26.8375, 101.75) ccw
  line L243 (-26.3375, 101.75) -> (-26.3375, 88.75)
  arc A244 (-174.475, 31.1) -> (-173.975, 31.6) centre (-174.475, 31.6) ccw
  line L244 (-174.475, 31.1) -> (-187.475, 31.1)
  arc A245 (-187.975, 31.6) -> (-187.475, 31.1) centre (-187.475, 31.6) ccw
  line L245 (-187.975, 31.6) -> (-187.975, 44.6)
  arc A246 (-187.475, 45.1) -> (-187.975, 44.6) centre (-187.475, 44.6) ccw
  line L246 (-187.475, 45.1) -> (-174.475, 45.1)
  arc A247 (-173.975, 44.6) -> (-174.475, 45.1) centre (-174.475, 44.6) ccw
  line L247 (-173.975, 44.6) -> (-173.975, 31.6)
  arc A248 (-260.2, 31.1) -> (-259.7, 31.6) centre (-260.2, 31.6) ccw
  line L248 (-260.2, 31.1) -> (-273.2, 31.1)
  arc A249 (-273.7, 31.6) -> (-273.2, 31.1) centre (-273.2, 31.6) ccw
  line L249 (-273.7, 31.6) -> (-273.7, 44.6)
  arc A250 (-273.2, 45.1) -> (-273.7, 44.6) centre (-273.2, 44.6) ccw
  line L250 (-273.2, 45.1) -> (-260.2, 45.1)
  arc A251 (-259.7, 44.6) -> (-260.2, 45.1) centre (-260.2, 44.6) ccw
  line L251 (-259.7, 44.6) -> (-259.7, 31.6)
  arc A252 (-212.575, 2.525) -> (-212.075, 3.025) centre (-212.575, 3.025) ccw
  line L252 (-212.575, 2.525) -> (-225.575, 2.525)
  arc A253 (-226.075, 3.025) -> (-225.575, 2.525) centre (-225.575, 3.025) ccw
  line L253 (-226.075, 3.025) -> (-226.075, 16.025)
  arc A254 (-225.575, 16.525) -> (-226.075, 16.025) centre (-225.575, 16.025) ccw
  line L254 (-225.575, 16.525) -> (-212.575, 16.525)
  arc A255 (-212.075, 16.025) -> (-212.575, 16.525) centre (-212.575, 16.025) ccw
  line L255 (-212.075, 16.025) -> (-212.075, 3.025)
  arc A256 (-217.3375, 88.25) -> (-216.8375, 88.75) centre (-217.3375, 88.75) ccw
  line L256 (-217.3375, 88.25) -> (-230.3375, 88.25)
  arc A257 (-230.8375, 88.75) -> (-230.3375, 88.25) centre (-230.3375, 88.75) ccw
  line L257 (-230.8375, 88.75) -> (-230.8375, 101.75)
  arc A258 (-230.3375, 102.25) -> (-230.8375, 101.75) centre (-230.3375, 101.75) ccw
  line L258 (-230.3375, 102.25) -> (-217.3375, 102.25)
  arc A259 (-216.8375, 101.75) -> (-217.3375, 102.25) centre (-217.3375, 101.75) ccw
  line L259 (-216.8375, 101.75) -> (-216.8375, 88.75)
  arc A260 (-79.225, 31.1) -> (-78.725, 31.6) centre (-79.225, 31.6) ccw
  line L260 (-79.225, 31.1) -> (-92.225, 31.1)
  arc A261 (-92.725, 31.6) -> (-92.225, 31.1) centre (-92.225, 31.6) ccw
  line L261 (-92.725, 31.6) -> (-92.725, 44.6)